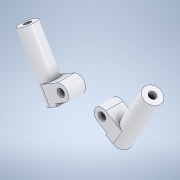
# Autodesk Inventor part: GripperCompensatorLeft
Saved by Autodesk Inventor 2021 (Build 250183000, 183)
## iProperties
Created: 2020-03-14
Part Number: GripperCompensatorLeft
Material: Generisch
Document SubType Name: Modeling
Designer: JochenAlt
Density: 1 g/cm^3
Appearance: Vorgabe
Author: JochenAlt
Autodesk Inventor part; units mm, degrees
ref_plane "YZ Plane" through (0, 0, 0) normal (1, 0, 0) x (0, 1, 0)
ref_plane "XZ Plane" through (0, 0, 0) normal (0, 1, 0) x (-1, 0, 0)
ref_plane "XY Plane" through (0, 0, 0) normal (0, 0, 1) x (1, 0, 0)
derived "Centre.ipt"
sketch "MainConstruction" plane through (0, 0, 0) normal (0, 0, 1) x (1, 0, 0)
  line L0 (-44.4573, 0) -> (45.9096, 0) construction
  line L1 (0, -41.3) -> (0, 41.3) construction
  line L2 (-12, 16.3923) -> (12, 16.3923) construction
  line L3 (20.547, 2.8038) -> (8.1962, -18.5885) construction
  line L4 (-8.1962, -18.5885) -> (-11.1962, -13.3923) construction
  line L5 (0, -16.3923) -> (24, -16.3923) construction
  line L6 (0, -16.3923) -> (-24, -16.3923) construction
  line L7 (6, -16.3923) -> (6, -10.3923) construction
  line L8 (6, -10.3923) -> (11.1962, -13.3923) construction
  line L9 (8.1962, -18.5885) -> (11.1962, -13.3923) construction
  line L10 (0, -16.3923) -> (6, -16.3923) construction
  line L11 (-6, -10.3923) -> (-6, -16.3923) construction
  line L12 (-6, -10.3923) -> (-11.1962, -13.3923) construction
  line L13 (0, 16.3923) -> (0, 0) construction
  line L14 (0, 0) -> (0, -16.3923) construction
  line L15 (-12, 14.3923) -> (12, 14.3923) construction
  line L16 (-12, 16.3923) -> (-12, 14.3923) construction
  line L17 (-12, 27) -> (12, 27) construction
  line L18 (-29.3827, -3.1077) -> (-17.3827, -23.8923) construction
  line L19 (0, 16.3923) -> (0, 27) construction
  line L20 (-23.3827, -13.5) -> (-14.1962, -8.1962) construction
  arc A0 (-2.6277, -14.0839) -> (-3.3698, -6.14) centre (-6, -10.3923) ccw construction
  arc A1 (3.3698, -6.14) -> (2.6277, -14.0839) centre (6, -10.3923) ccw construction
  line L21 (-27.2176, -1.8577) -> (-31.5477, -4.3577) construction
  line L22 (-15.2176, -22.6423) -> (-19.5477, -25.1423) construction
  line L23 (19.5477, -25.1423) -> (15.2176, -22.6423) construction
  circle A2 centre (0, 0) radius 22 construction
  line L24 (12, 14.3923) -> (12, 16.3923) construction
  line L25 (23.3827, -13.5) -> (14.1962, -8.1962) construction
  line L26 (20.1962, 2.1962) -> (14.1962, -8.1962) construction
  line L27 (11.1962, -13.3923) -> (14.1962, -8.1962) construction
  line L28 (-6, -16.3923) -> (0, -16.3923) construction
  line L29 (8.1962, -18.5885) -> (15.2176, -22.6423) construction
  line L30 (-15.2176, -22.6423) -> (-8.1962, -18.5885) construction
  line L31 (-12, 29.5) -> (-12, 24.5) construction
  line L32 (12, 29.5) -> (12, 24.5) construction
  line L33 (12, 24.5) -> (12, 16.3923) construction
  line L34 (-12, 24.5) -> (-12, 16.3923) construction
  line L35 (-11.1962, -13.3923) -> (-8.1962, -18.5885) construction
  line L36 (-11.1962, -13.3923) -> (-20.1962, 2.1962) construction
  line L37 (27.2176, -1.8577) -> (31.5477, -4.3577) construction
  line L38 (17.3827, -23.8923) -> (29.3827, -3.1077) construction
  line L39 (27.2176, -1.8577) -> (21.9687, 1.1728) construction
  line L40 (-27.2176, -1.8577) -> (-21.9687, 1.1728) construction
  line L41 (20.1962, 2.1962) -> (21.9687, 1.1728) construction
  line L42 (-21.9687, 1.1728) -> (-20.1962, 2.1962) construction
  line L43 (0, -16.3923) -> (0, -24.5) construction
  line L44 (0, -24.5) -> (0, -29.5) construction
  line L45 (0, -27) -> (24, -27) construction
  line L46 (18.4641, 3.1962) -> (6.4641, -17.5885) construction
  line L47 (-18.4641, 3.1962) -> (-6.4641, -17.5885) construction
  line L48 (-20.1962, 2.1962) -> (-18.4641, 3.1962) construction
  line L49 (20.1962, 2.1962) -> (18.4641, 3.1962) construction
  line L50 (3.3698, -6.14) -> (18.4641, 3.1962) construction
  line L51 (-18.4641, 3.1962) -> (-3.3698, -6.14) construction
  circle A3 centre (30.5, 27) radius 2.5 construction
  line L52 (12, 14.3923) -> (16.25, 14.3923) construction
  line L53 (16.25, 14.3923) -> (31.8962, 24.9262) construction
  line L54 (29.1038, 29.0738) -> (10.2677, 16.3923) construction
  line L55 (12, 16.3923) -> (10.2677, 16.3923) construction
  line L56 (8.1962, -18.5885) -> (6.4641, -17.5885) construction
  line L57 (6.4641, -17.5885) -> (2.6277, -14.0839) construction
  line L58 (-8.1962, -18.5885) -> (-6.4641, -17.5885) construction
  line L59 (-6.4641, -17.5885) -> (-2.6277, -14.0839) construction
sketch "Skizze2" plane through (0, 0, 0) normal (0, 0, 1) x (1, 0, 0)
  line L0 (-44.4573, 0) -> (45.9096, 0) construction
  line L1 (0, -41.3) -> (0, 41.3) construction
  line L2 (20.547, 2.8038) -> (8.1962, -18.5885) construction
  line L3 (-12, 16.3923) -> (12, 16.3923) construction
  line L4 (0, -16.3923) -> (24, -16.3923) construction
  line L5 (0, -16.3923) -> (-24, -16.3923) construction
  circle A0 centre (-6, -10.3923) radius 1.1
  arc A1 (-4.875, -12.3409) -> (-7.125, -8.4437) centre (-6, -10.3923) ccw
  line L6 (-16.0981, 1.0981) -> (-20.4282, -1.4019)
  line L7 (-16.0981, 1.0981) -> (-7.4731, -13.8409)
  line L8 (-20.4282, -1.4019) -> (-14.0532, -12.4437)
  line L9 (-7.125, -8.4437) -> (-14.0532, -12.4437)
  arc A2 (-7.9486, -11.5173) -> (-4.875, -12.3409) centre (-6, -10.3923) ccw
  line L10 (-14.0532, -12.4437) -> (-12.0108, -15.9812)
  line L11 (-23.3827, -13.5) -> (-14.1962, -8.1962) construction
  line L12 (-12.0108, -15.9812) -> (-11.4282, -16.9904)
  line L13 (-7.4731, -13.8409) -> (-7.0981, -14.4904)
  line L14 (-7.0981, -14.4904) -> (-11.4282, -16.9904)
  line L15 (-7.4731, -13.8409) -> (-4.875, -12.3409)
  line L16 (-7.4731, -13.8409) -> (-11.8032, -16.3409)
  arc A3 (-7.125, -8.4437) -> (-7.9486, -11.5173) centre (-6, -10.3923) ccw
  line L17 (-29.3827, -3.1077) -> (-17.3827, -23.8923) construction
  line L18 (-11.1962, -13.3923) -> (-20.1962, 2.1962) construction
  line L19 (-18.2631, -0.1519) -> (-9.2631, -15.7404) construction
  point P0 (0, 0)
  point P1 (6, -10.3923)
  point P2 (-9.6962, -15.9904)
  point P3 (-9.2274, -9.6576)
  point P4 (-9.7231, -9.9437)
  point P5 (-6.9774, -13.5547)
  dimension "d1" = 2.2
  dimension "d2" = 4.5
  dimension "d31" = 5
  dimension "d41" = 3
  dimension "d43" = 5.5
  constraints: 23 end point, 7 point on circle, 6 perpendicular, 4 centre point, 4 point on line, 3 coincident, 2 collinear, 2 midpoint, 2 parallel, 2 tangent, 1 concentric, 1 other
  measures "d1" diameter of A0
  measures "d2" diameter of A1
  measures "d31" distance of L6.start L6.end
  measures "d41" distance from line of L6 L18.end
  measures "d43" distance from line of A1.centre L19
extrude "Extrusion6" add sketch "Skizze2" along normal blind 5
sketch "Profile" plane through (-18.9282, -0.5359, 0.25) normal (-0.5, 0.8660254, 0) x (0.8660254, 0.5, 0)
  circle A0 centre (0.7679, -2.25) radius 2.5
  circle A1 centre (0.7679, -2.25) radius 1
  line L0 (0.7679, 0.25) -> (0, 0.25)
  line L1 (3.2679, 0.25) -> (3.2679, -4.75) projected
  line L2 (-1.7321, 0.25) -> (-1.7321, -4.75) projected
  line L3 (3.2679, -4.75) -> (-1.7321, -4.75) projected
  line L4 (3.2679, 0.25) -> (-1.7321, 0.25) projected
  line L5 (-1.7321, 0.25) -> (-1.7321, -4.75) projected
  line L6 (-1.7321, -4.75) -> (3.2679, -4.75)
  point P0 (16.6603, 0.25)
  point P1 (-1.7321, -4.75)
  dimension "d12" = 2
  constraints: 4 end point, 4 horizontal, 2 point on line, 2 vertical, 1 centre point, 1 coincident, 1 vertical alignment, 2 other
  measures "d12" diameter of A1
extrude "Extrusion3" cut sketch "Profile" against normal through all contours A1
fillet "Rundung1" radius 2.5 5 edges at (-12.9106, -4.4228, 0) (-7.2856, -14.1656, 0) (-15.9282, -9.1962, 5) (-15.9282, -9.1962, 0) (-12.9106, -4.4228, 5)
mirror "Spiegeln1" about plane through (0, 0, 0) normal (1, 0, 0) bodies 1 separate body
